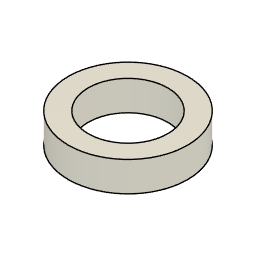
Spacer φ8.0 x 3.0mm (Autodesk Fusion 360 design; units mm, degrees)
Autodesk Fusion 360 part; units mm, degrees
sketch "スケッチ1" plane through (0, 0, 0) normal (0, 1, 0) x (1, 0, 0)
  circle A0 centre (0, 0) radius 6
  dimension "d1" = 12
  constraint coincident A0.centre origin
  measures "d1" diameter of A0
extrude "押し出し1" add sketch "スケッチ1" along normal blind 3.7
sketch "スケッチ2" plane through (0, 3.7, 0) normal (0, 1, 0) x (-1, 0, 0)
  circle A0 centre (0, 0) radius 6
  constraint coincident A0.centre origin
hole "穴1" at (0, 3.7, 0) direction (0, -1, 0) diameter 8 depth 10 tip angle 118
extrude "押し出し2" add 1 faces at (5.3073, 3.7, 0.3977) along direction (0, 1, 0) blind 1
sketch "スケッチ3" plane through (0, 4.7, 0) normal (0, 1, 0) x (-1, 0, 0)
  circle A0 centre (0, 0) radius 4
  circle A1 centre (0, 0) radius 6
  circle A2 centre (0, 0) radius 13.5
  dimension "d9" = 27
  constraint coincident A0.centre A1.centre
  measures "d9" diameter of A2
extrude "押し出し3" add sketch "スケッチ3" along normal blind 2 contours A1 | A2
extrude "押し出し4" cut 1 faces at (-10.2682, 6.7, -0.8694) along direction (0, -1, 0) blind 2
extrude "押し出し5" cut 1 faces at (5.3073, 4.7, 0.3977) along direction (0, -1, 0) blind 1.7
